# Autodesk Inventor part: GESTURESENSE_LOGOSTEXT
Saved by Autodesk Inventor 2016 SP1 (Build 200210100, 210)
## iProperties
Created: 2015-11-19
Part Number: GESTURESENSE_LOGOSTEXT
Material: Generic
Document SubType Name: Modeling
Designer: PhillipD
Density: 1 g/cm^3
Appearance: GESTURESENSE_TEXT, GESTURESENSE_LOGOSTEXT
Author: PhillipD
Autodesk Inventor part; units mm, degrees
ref_plane "YZ Plane" through (0, 0, 0) normal (1, 0, 0) x (0, 1, 0)
ref_plane "XZ Plane" through (0, 0, 0) normal (0, 1, 0) x (-1, 0, 0)
ref_plane "XY Plane" through (0, 0, 0) normal (0, 0, 1) x (1, 0, 0)
sketch "GESTURESENSE_TEXT, GESTURESENSE_LOGOSTEXT_67" plane through (0, 0, 0) normal (0, 0, 1) x (1, 0, 0)
  line L0 (0, 7.52) -> (11.51, 7.52)
  line L1 (11.51, 7.52) -> (11.51, 0)
  line L2 (11.51, 0) -> (0, 0)
  line L3 (0, 0) -> (0, 7.52)
  constraints: 8 end point
extrude "Extrusion1" add sketch "GESTURESENSE_TEXT, GESTURESENSE_LOGOSTEXT_67" along normal blind 1
body "Solid1"
